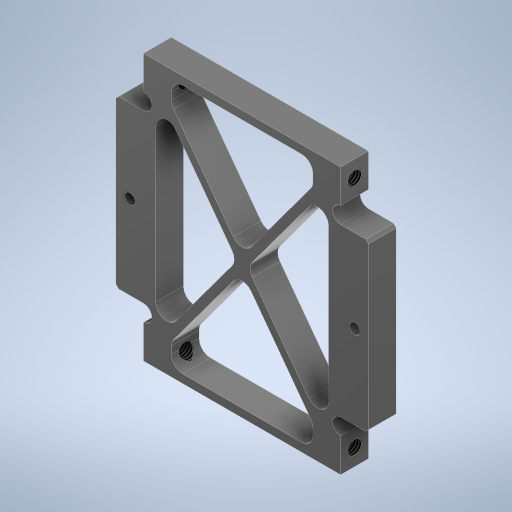
# Autodesk Inventor part: KneeBraceFrame
Saved by Autodesk Inventor 2024.2 (Build 282272000, 272)
## iProperties
Created: 2024-01-11
Part Number: KneeBraceFrame
Material: Acetal Resin, Black
Document SubType Name: Modeling
Designer: Masato Kubotera
Density: 1.425 g/cm^3
Appearance: Smooth - Black
Vendor: meviy
Mass: 5.52818 g
Surface Area: 42.1146 cm^2
Volume: 3.87943 cm^3
Author: Masato Kubotera
Autodesk Inventor part; units mm, degrees
ref_plane "YZ Plane" through (0, 0, 0) normal (1, 0, 0) x (0, 1, 0)
ref_plane "XZ Plane" through (0, 0, 0) normal (0, 1, 0) x (-1, 0, 0)
ref_plane "XY Plane" through (0, 0, 0) normal (0, 0, 1) x (1, 0, 0)
sketch "Sketch1" plane through (0, 0, 0) normal (1, 0, 0) x (0, 1, 0)
  line L0 (-17.75, 24) -> (17.75, 24)
  line L1 (17.75, 24) -> (17.75, -24)
  line L2 (17.75, -24) -> (-17.75, -24)
  line L3 (-17.75, -24) -> (-17.75, 24)
  line L4 (-17.75, 24) -> (17.75, -24) construction
  line L5 (17.75, 24) -> (-17.75, -24) construction
  line L6 (17.75, 15) -> (22.75, 15)
  line L7 (22.75, 15) -> (22.75, -15)
  line L8 (22.75, -15) -> (17.75, -15)
  line L9 (17.75, 0) -> (-17.75, 0) construction
  line L10 (0, 24) -> (0, -24)
  arc A0 (17.75, 18) -> (17.75, 15) centre (17.75, 16.5) ccw
  line L11 (17.75, -15) -> (22.75, -15)
  arc A1 (17.75, -15) -> (17.75, -18) centre (17.75, -16.5) ccw
  line L12 (-17.75, 15) -> (-22.75, 15)
  line L13 (-22.75, 15) -> (-22.75, -15)
  line L14 (-22.75, -15) -> (-17.75, -15)
  arc A2 (-17.75, 15) -> (-17.75, 18) centre (-17.75, 16.5) ccw
  arc A3 (-17.75, -18) -> (-17.75, -15) centre (-17.75, -16.5) ccw
  line L15 (17.75, 21) -> (12.75, 21) construction
  line L16 (-10.75, 22.5) -> (10.75, 22.5)
  line L17 (12.358, 17.9707) -> (1.608, 3.4355)
  line L18 (-12.358, 17.9707) -> (-1.608, 3.4355)
  line L19 (1.8124, 1.1893) -> (11.9735, 14.9282)
  line L20 (15.5815, 13.7389) -> (15.5815, -13.7389)
  line L21 (1.8124, -1.1893) -> (11.9735, -14.9282)
  arc A4 (-1.608, 3.4355) -> (1.608, 3.4355) centre (0, 4.6248) ccw
  arc A5 (15.5815, 13.7389) -> (11.9735, 14.9282) centre (13.5815, 13.7389) ccw
  arc A6 (1.8124, 1.1893) -> (1.8124, -1.1893) centre (3.4204, 0) ccw
  arc A7 (11.9735, -14.9282) -> (15.5815, -13.7389) centre (13.5815, -13.7389) ccw
  line L22 (17.75, -21) -> (12.75, -21) construction
  line L23 (12.75, 19.16) -> (12.75, 20.5)
  line L24 (-12.75, 19.16) -> (-12.75, 20.5)
  arc A8 (12.75, 20.5) -> (10.75, 22.5) centre (10.75, 20.5) ccw
  arc A9 (12.358, 17.9707) -> (12.75, 19.16) centre (10.75, 19.16) ccw
  arc A10 (-10.75, 22.5) -> (-12.75, 20.5) centre (-10.75, 20.5) ccw
  arc A11 (-12.75, 19.16) -> (-12.358, 17.9707) centre (-10.75, 19.16) ccw
  circle A12 centre (20.25, 0) radius 1 construction
  line L25 (20.25, 15) -> (20.25, -15) construction
  line L26 (-10.75, -22.5) -> (10.75, -22.5)
  line L27 (12.358, -17.9707) -> (1.608, -3.4355)
  line L28 (-12.358, -17.9707) -> (-1.608, -3.4355)
  arc A13 (1.608, -3.4355) -> (-1.608, -3.4355) centre (0, -4.6248) ccw
  line L29 (12.75, -19.16) -> (12.75, -20.5)
  line L30 (-12.75, -19.16) -> (-12.75, -20.5)
  arc A14 (10.75, -22.5) -> (12.75, -20.5) centre (10.75, -20.5) ccw
  arc A15 (12.75, -19.16) -> (12.358, -17.9707) centre (10.75, -19.16) ccw
  arc A16 (-12.75, -20.5) -> (-10.75, -22.5) centre (-10.75, -20.5) ccw
  arc A17 (-12.358, -17.9707) -> (-12.75, -19.16) centre (-10.75, -19.16) ccw
  point P0 (0, 0)
  point P1 (0, 1.2613)
  point P2 (0.9328, 0)
  point P3 (15.5815, 19.8066)
  point P4 (15.5815, -19.8066)
  point P5 (-12.75, 22.5)
  point P6 (12.75, 22.5)
  point P7 (0, 2.6248)
  point P8 (17.75, -18)
  point P9 (0, 22.5)
  point P10 (12.75, 18.5007)
  point P11 (-12.75, 18.5007)
  point P12 (0, -2.6248)
  point P13 (0, -22.5)
  dimension "d0" = 1.5
  dimension "d1" = 5
  dimension "d2" = 48
  dimension "d3" = 9
  dimension "d4" = 35.5
  dimension "d5" = 5
  dimension "d6" = 1.5
  dimension "d8" = 1.5
  dimension "d9" = 1.5
  dimension "d22" = 2
  dimension "d24" = 2
  constraints: 62 end point, 34 point on circle, 31 symmetric about line, 28 point on line, 18 centre point, 16 tangent, 9 midpoint, 7 equal radius, 4 horizontal, 3 parallel, 3 vertical, 1 coincident, 1 perpendicular, 11 other
  measures "d0" radius of A0
  measures "d1" distance of L6.start L6.end
  measures "d2" distance between parallel lines of L2 L0
  measures "d3" distance of L6.start L0.end
  measures "d4" distance of L0.start L0.end
  measures "d5" distance of L15.start L15.end
  measures "d6" distance between parallel lines of L16 L0
  measures "d8" distance between parallel lines of L19 L17
  measures "d22" radius of A5
  measures "d24" diameter of A12
extrude "Extrusion1" add sketch "Sketch1" along normal blind 5 contours L0 L1 A0 A1 L2 L10 L26 A14 L29 A15 L27 A13 A4 L17 A9 L23 A8 L16 | L6 L7 L8 L1
sketch "Sketch2" plane through (0, 17.75, 24) normal (0, 1, 0) x (1, 0, 0)
  line L0 (0, 45) -> (5, 45)
  line L1 (0, 3) -> (5, 3)
  line L2 (5, 6) -> (5, 0) projected
  line L3 (5, 48) -> (5, 42) projected
  line L4 (0, 6) -> (0, 0) projected
  line L5 (0, 48) -> (0, 42) projected
  point P0 (0, 3)
  point P1 (0, 3)
  point P2 (0, 3)
  point P3 (0, 45)
  point P4 (2.5, 3)
  point P5 (2.5, 45)
  constraints: 6 midpoint, 4 end point, 2 horizontal
hole "Side-M3" at (2.5, 17.75, -21) at (2.5, 17.75, 21) direction (0, -1, 0) diameter 2.459 end through all thread size "M3x0.5" class "6H" standard "ISO Metric profile"
hole "Phi2-H7" at (0, 20.25, 0) direction (1, 0, 0) diameter 2 end through all
chamfer "C0.5" distance 0.5 angle 45 2 edges at (2.5, 22.75, 15) (2.5, 22.75, -15)
mirror "Mirror1" about plane through (0, 0, 2.6248) normal (0, -1, 0)
equation "\"d8\" = d6"
equation "\"d9\" = d6"
equation "\"d17\" = d5"
body "Solid1"
